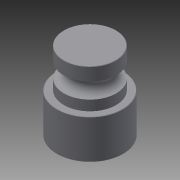
# Autodesk Inventor part: slik_clamp_head38_stud
Saved by Autodesk Inventor 2013 (Build 170138000, 138)
## iProperties
Created: 2013-01-30
Part Number: slik_clamp_head38_stud
Material: Generic
Document SubType Name: Modeling
Designer: Mahisorn
Density: 1 g/cm^3
Author: Mahisorn
Autodesk Inventor part; units mm, degrees
ref_plane "YZ Plane" through (0, 0, 0) normal (1, 0, 0) x (0, 1, 0)
ref_plane "XZ Plane" through (0, 0, 0) normal (0, 1, 0) x (-1, 0, 0)
ref_plane "XY Plane" through (0, 0, 0) normal (0, 0, 1) x (1, 0, 0)
sketch "Sketch1" plane through (0, 0, 0) normal (0, 0, 1) x (1, 0, 0)
  line L0 (0, 0) -> (0, 20)
  line L1 (0, 20) -> (13.45, 20)
  line L2 (13.45, 20) -> (13.45, 13.2)
  line L3 (0, 0) -> (13.45, 0)
  line L4 (13.45, 0) -> (13.45, 5.2)
  arc A0 (13.45, 13.2) -> (13.45, 5.2) centre (13.45, 9.2) ccw
  dimension "d0" = 20
  dimension "d1" = 13.45
  dimension "d2" = 6.8
  dimension "d3" = 13.45
  dimension "d4" = 8
  dimension "d5" = 4
  constraints: 10 end point, 4 perpendicular, 2 point on circle, 1 centre point, 1 vertical
  measures "d0" distance of L0.start L0.end
  measures "d1" distance of L0.end L1.end
  measures "d2" distance of L1.end L2.end
  measures "d3" distance of L0.start L3.end
  measures "d4" distance of L4.end L2.end
  measures "d5" radius of A0
revolve "Revolution1" add sketch "Sketch1" angle 360 about axis through (0, 0, 0) along (0, 1, 0)
chamfer "Chamfer1" distance 0.2 angle 45 1 edges at (-13.45, 20, 0)
sketch "Sketch2" plane through (0, 0, 0) normal (0, -1, 0) x (1, 0, 0)
  circle A0 centre (0, 0) radius 13.45 projected
  circle A1 centre (0, 0) radius 17
  dimension "d10" = 34
  constraints: 1 centre point, 1 coincident
  measures "d10" diameter of A1
extrude "Extrusion1" add sketch "Sketch2" along normal blind 20 contours A0 | A1
chamfer "Chamfer2" distance 0.2 angle 45 1 edges at (-17, 0, 0)
body "Solid1"
